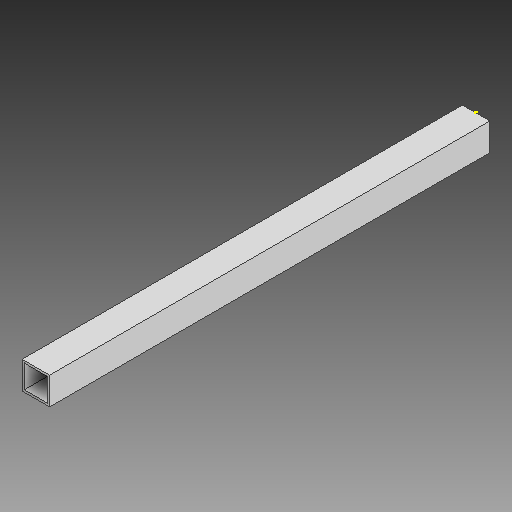
# Autodesk Inventor part: SteherStrebe
Saved by Autodesk Inventor 2021 (Build 250183000, 183)
## iProperties
Created: 2021-09-01
Part Number: SteherStrebe
Material: Generisch
Document SubType Name: Modeling
Designer: lukas
Density: 1 g/cm^3
Appearance: Vorgabe
Stock Number: Steher Strebe
Author: lukas
Autodesk Inventor part; units mm, degrees
ref_plane "YZ Plane" through (0, 0, 0) normal (1, 0, 0) x (0, 1, 0)
ref_plane "XZ Plane" through (0, 0, 0) normal (0, 1, 0) x (-1, 0, 0)
ref_plane "XY Plane" through (0, 0, 0) normal (0, 0, 1) x (1, 0, 0)
sketch "Skizze2" plane through (0, 0, 0) normal (0, 0, 1) x (1, 0, 0)
  line L0 (-17.5, 0) -> (17.5, 0) projected
  line L1 (0, -17.5) -> (0, 17.5) projected
  line L2 (-12.5, 12.5) -> (12.5, 12.5)
  line L3 (12.5, 12.5) -> (12.5, -12.5)
  line L4 (12.5, -12.5) -> (-12.5, -12.5)
  line L5 (-12.5, -12.5) -> (-12.5, 12.5)
  point P0 (0, 0)
  dimension "d3" = 25
  dimension "d4" = 25
  constraints: 8 end point, 2 parallel, 1 horizontal, 1 perpendicular, 2 other
  measures "d3" distance of L3.end L4.end
  measures "d4" distance between parallel lines of L2 L4
extrude "Extrusion2" add sketch "Skizze2" along normal blind 400
sketch "Skizze3" plane through (-12.5, 12.5, 0) normal (0, 1, 0) x (1, 0, 0)
  point P0 (12.5, 0)
sketch "Skizze4" plane through (0, 0, 400) normal (0, 0, 1) x (1, 0, 0)
  line L0 (-10.5, -10.5) -> (10.5, -10.5)
  line L1 (10.5, -10.5) -> (10.5, 10.5)
  line L2 (10.5, 10.5) -> (-10.5, 10.5)
  line L3 (-10.5, 10.5) -> (-10.5, -10.5)
  line L4 (-12.5, 12.5) -> (-12.5, -12.5) projected
  line L5 (12.5, 12.5) -> (-12.5, 12.5) projected
  line L6 (12.5, -12.5) -> (12.5, 12.5) projected
  line L7 (-12.5, -12.5) -> (12.5, -12.5) projected
  point P0 (0, 0)
  dimension "d7" = 2
  dimension "d8" = 2
  dimension "d9" = 2
  dimension "d10" = 2
  constraints: 8 end point, 2 parallel, 1 horizontal, 1 perpendicular
  measures "d7" distance between parallel lines of L4 L3
  measures "d8" distance between parallel lines of L5 L2
  measures "d9" distance between parallel lines of L6 L1
  measures "d10" distance between parallel lines of L7 L0
extrude "Extrusion3" cut sketch "Skizze4" against normal blind 500 contours L3 L2 L1 L0
